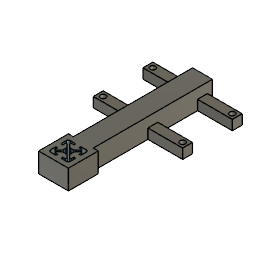
Spiegel Houder (Autodesk Fusion 360 design; units mm, degrees)
part number: 2026-06-02-17-48-06-429
Autodesk Fusion 360 part; units mm, degrees
note: some values were not read from the file. Set by a fixed rule: which sketch regions a step uses.
sketch "Item profile" plane through (0, 0, 0) normal (0, 0, 1) x (1, 0, 0)
  line L0 (2.5199, -9.1957) -> (2.5199, -8.4981)
  spline S0 degree 3 poles (2.5199, -8.4981) (2.5279, -8.3313) (2.6117, -8.22) (2.8181, -8.1997) knots 0 0 0 0 1 1 1 1
  line L1 (2.8181, -8.1997) -> (4.9343, -8.1997)
  spline S1 degree 3 poles (4.9343, -8.1997) (5.7717, -8.1578) (5.9819, -7.2415) (5.5227, -6.7803) knots 0 0 0 0 1 1 1 1
  line L2 (5.5227, -6.7803) -> (3.2736, -4.5302)
  spline S2 degree 3 poles (3.2736, -4.5302) (2.3958, -3.7139) (1.5457, -3.6474) (1.1575, -3.6552) knots 0 0 0 0 1 1 1 1
  line L3 (1.1575, -3.6552) -> (-1.1199, -3.6552)
  spline S3 degree 3 poles (-1.1199, -3.6552) (-1.5201, -3.6474) (-2.3702, -3.7139) (-3.2481, -4.5302) knots 0 0 0 0 1 1 1 1
  line L4 (-3.2481, -4.5302) -> (-5.4972, -6.7803)
  spline S4 degree 3 poles (-5.4972, -6.7803) (-5.9564, -7.2415) (-5.7462, -8.1578) (-4.9087, -8.1997) knots 0 0 0 0 1 1 1 1
  line L5 (-4.9087, -8.1997) -> (-2.7926, -8.1997)
  spline S5 degree 3 poles (-2.7926, -8.1997) (-2.5862, -8.22) (-2.5027, -8.3313) (-2.4943, -8.4981) knots 0 0 0 0 1 1 1 1
  line L6 (-2.4943, -8.4981) -> (-2.4943, -9.1957)
  spline S6 degree 3 poles (-2.4943, -9.1957) (-2.5003, -9.6292) (-2.8228, -9.9778) (-3.2985, -9.9941) knots 0 0 0 0 1 1 1 1
  line L7 (-3.2985, -9.9941) -> (-7.9963, -9.9941)
  spline S7 degree 3 poles (-7.9963, -9.9941) (-9.0202, -10.009) (-10.0068, -9.1289) (-9.9915, -7.994) knots 0 0 0 0 1 1 1 1
  line L8 (-9.9915, -7.994) -> (-9.9915, -3.3004)
  spline S8 degree 3 poles (-9.9915, -3.3004) (-9.9752, -2.8306) (-9.6268, -2.5081) (-9.1934, -2.502) knots 0 0 0 0 1 1 1 1
  line L9 (-9.1934, -2.502) -> (-8.4961, -2.502)
  spline S9 degree 3 poles (-8.4961, -2.502) (-8.3294, -2.5103) (-8.2182, -2.5938) (-8.1978, -2.8003) knots 0 0 0 0 1 1 1 1
  line L10 (-8.1978, -2.8003) -> (-8.1978, -4.9173)
  spline S10 degree 3 poles (-8.1978, -4.9173) (-8.1559, -5.7552) (-7.24, -5.9654) (-6.779, -5.5061) knots 0 0 0 0 1 1 1 1
  line L11 (-6.779, -5.5061) -> (-4.5299, -3.256)
  spline S11 degree 3 poles (-4.5299, -3.256) (-3.7139, -2.3778) (-3.6474, -1.5274) (-3.6552, -1.139) knots 0 0 0 0 1 1 1 1
  line L12 (-3.6552, -1.139) -> (-3.6552, 1.1393)
  spline S12 degree 3 poles (-3.6552, 1.1393) (-3.6472, 1.5397) (-3.7138, 2.3901) (-4.5299, 3.2683) knots 0 0 0 0 1 1 1 1
  line L13 (-4.5299, 3.2683) -> (-6.779, 5.5184)
  spline S13 degree 3 poles (-6.779, 5.5184) (-7.24, 5.9777) (-8.1559, 5.7675) (-8.1978, 4.9297) knots 0 0 0 0 1 1 1 1
  line L14 (-8.1978, 4.9297) -> (-8.1978, 2.8127)
  spline S14 degree 3 poles (-8.1978, 2.8127) (-8.2181, 2.6062) (-8.3294, 2.5226) (-8.4961, 2.5143) knots 0 0 0 0 1 1 1 1
  line L15 (-8.4961, 2.5143) -> (-9.1934, 2.5143)
  spline S15 degree 3 poles (-9.1934, 2.5143) (-9.6267, 2.5204) (-9.9752, 2.8429) (-9.9915, 3.3085) knots 0 0 0 0 1 1 1 1
  line L16 (-9.9915, 3.3085) -> (-9.9915, 7.9981)
  spline S16 degree 3 poles (-9.9915, 7.9981) (-10.0064, 9.0224) (-9.1267, 10.0093) (-7.9922, 9.9941) knots 0 0 0 0 1 1 1 1
  line L17 (-7.9922, 9.9941) -> (-3.3005, 9.9941)
  spline S17 degree 3 poles (-3.3005, 9.9941) (-2.8309, 9.9778) (-2.5086, 9.6292) (-2.5024, 9.1957) knots 0 0 0 0 1 1 1 1
  line L18 (-2.5024, 9.1957) -> (-2.5024, 8.4981)
  spline S18 degree 3 poles (-2.5024, 8.4981) (-2.5104, 8.3313) (-2.5943, 8.22) (-2.8007, 8.1997) knots 0 0 0 0 1 1 1 1
  line L19 (-2.8007, 8.1997) -> (-4.9168, 8.1997)
  spline S19 degree 3 poles (-4.9168, 8.1997) (-5.7543, 8.1578) (-5.9645, 7.2415) (-5.5053, 6.7803) knots 0 0 0 0 1 1 1 1
  line L20 (-5.5053, 6.7803) -> (-3.2562, 4.5302)
  spline S20 degree 3 poles (-3.2562, 4.5302) (-2.3783, 3.7139) (-1.5283, 3.6474) (-1.14, 3.6552) knots 0 0 0 0 1 1 1 1
  line L21 (-1.14, 3.6552) -> (1.1373, 3.6552)
  spline S21 degree 3 poles (1.1373, 3.6552) (1.5376, 3.6474) (2.3877, 3.7139) (3.2655, 4.5302) knots 0 0 0 0 1 1 1 1
  line L22 (3.2655, 4.5302) -> (5.5147, 6.7803)
  spline S22 degree 3 poles (5.5147, 6.7803) (5.9738, 7.2414) (5.7636, 8.1577) (4.9262, 8.1996) knots 0 0 0 0 1 1 1 1
  line L23 (4.9262, 8.1996) -> (2.81, 8.1996)
  spline S23 degree 3 poles (2.81, 8.1996) (2.6036, 8.22) (2.5201, 8.3312) (2.5118, 8.498) knots 0 0 0 0 1 1 1 1
  line L24 (2.5118, 8.498) -> (2.5118, 9.1956)
  spline S24 degree 3 poles (2.5118, 9.1956) (2.5178, 9.6292) (2.8403, 9.9778) (3.3159, 9.994) knots 0 0 0 0 1 1 1 1
  line L25 (3.3159, 9.994) -> (8.0137, 9.9941)
  spline S25 degree 3 poles (8.0137, 9.9941) (9.0376, 10.009) (10.0242, 9.1289) (10.0089, 7.994) knots 0 0 0 0 1 1 1 1
  line L26 (10.0089, 7.994) -> (10.0089, 3.3004)
  spline S26 degree 3 poles (10.0089, 3.3004) (9.9927, 2.8306) (9.6442, 2.5081) (9.2109, 2.502) knots 0 0 0 0 1 1 1 1
  line L27 (9.2109, 2.502) -> (8.5136, 2.502)
  spline S27 degree 3 poles (8.5136, 2.502) (8.3468, 2.5103) (8.2356, 2.5938) (8.2153, 2.8003) knots 0 0 0 0 1 1 1 1
  line L28 (8.2153, 2.8003) -> (8.2153, 4.9173)
  spline S28 degree 3 poles (8.2153, 4.9173) (8.1734, 5.7551) (7.2575, 5.9654) (6.7965, 5.5061) knots 0 0 0 0 1 1 1 1
  line L29 (6.7965, 5.5061) -> (4.5473, 3.256)
  spline S29 degree 3 poles (4.5473, 3.256) (3.7313, 2.3778) (3.6649, 1.5274) (3.6727, 1.139) knots 0 0 0 0 1 1 1 1
  line L30 (3.6727, 1.139) -> (3.6727, -1.1392)
  spline S30 degree 3 poles (3.6727, -1.1392) (3.6646, -1.5397) (3.7312, -2.3901) (4.5473, -3.2683) knots 0 0 0 0 1 1 1 1
  line L31 (4.5473, -3.2683) -> (6.7964, -5.5184)
  spline S31 degree 3 poles (6.7964, -5.5184) (7.2574, -5.9777) (8.1734, -5.7675) (8.2153, -4.9296) knots 0 0 0 0 1 1 1 1
  line L32 (8.2153, -4.9296) -> (8.2153, -2.8126)
  spline S32 degree 3 poles (8.2153, -2.8126) (8.2356, -2.6061) (8.3468, -2.5226) (8.5135, -2.5143) knots 0 0 0 0 1 1 1 1
  line L33 (8.5135, -2.5143) -> (9.2108, -2.5143)
  spline S33 degree 3 poles (9.2108, -2.5143) (9.6442, -2.5204) (9.9927, -2.8429) (10.0089, -3.3127) knots 0 0 0 0 1 1 1 1
  line L34 (10.0089, -3.3127) -> (10.0089, -8.0063)
  spline S34 degree 3 poles (10.0089, -8.0063) (10.0242, -9.1412) (9.0376, -10.0213) (8.0137, -10.0064) knots 0 0 0 0 1 1 1 1
  line L35 (8.0137, -10.0064) -> (3.32, -10.0002)
  spline S35 degree 3 poles (3.32, -10.0002) (2.8483, -9.9778) (2.526, -9.6292) (2.5199, -9.1957) knots 0 0 0 0 1 1 1 1
  circle A0 centre (0, 0) radius 3.6552 construction
  constraint tangent L3 A0
  constraint tangent L12 A0
  constraint tangent L21 A0
  constraint coincident A0.centre origin
sketch "Body profile" plane through (0, 0, 0) normal (0, 0, 1) x (1, 0, 0)
  line L0 (15, 15) -> (-15, 15)
  line L1 (-15, 15) -> (-15, -15)
  line L2 (-15, -15) -> (15, -15)
  line L3 (15, -15) -> (15, 15)
  line L4 (15, 15) -> (-15, -15) construction
  line L5 (-15, 15) -> (15, -15) construction
  dimension "d1" = 30
  dimension "d2" = 30
  constraint horizontal L0
  constraint perpendicular L0 L1
  constraint parallel L0 L2
  constraint parallel L1 L3
  constraint coincident L4 origin
  constraint coincident L5 origin
  measures "d1" distance of L1.end L2.end
  measures "d2" distance of L0.end L1.end
extrude "Extrude1" add sketch "Body profile" along normal blind 20
extrude "Extrude13" cut sketch "Item profile" along normal blind 20
sketch "Sketch11" plane through (0, 15, 0) normal (0, 1, 0) x (1, 0, 0)
  line L0 (10, 0) -> (-10, 0) construction
  line L1 (10, 0) -> (-10, 0)
  line L2 (-10, 0) -> (-10, -20)
  line L3 (-10, -20) -> (10, -20)
  line L4 (10, -20) -> (10, 0)
  line L5 (15, 0) -> (-15, 0)
  line L6 (-15, 0) -> (-15, -20)
  line L7 (-15, -20) -> (15, -20)
  line L8 (15, -20) -> (15, 0)
  dimension "d60" = 20
  dimension "d61" = 20
  constraint horizontal L1
  constraint vertical L2
  constraint horizontal L3
  constraint vertical L4
  constraint coincident L0.start L1.start
  measures "d60" distance of L0.start L0.end
  measures "d61" distance of L0.start L3.end
extrude "Extrude9" add sketch "Sketch11" along normal blind 120 contours L1 L2 L3 L4 L5 L7
sketch "Sketch12" plane through (-10, 0, 0) normal (-1, 0, 0) x (0, -1, 0)
  line L0 (-15, 0) -> (-15, 20)
  line L1 (-130, 0) -> (-120, 0)
  line L2 (-120, 0) -> (-120, 10)
  line L3 (-120, 10) -> (-130, 10)
  line L4 (-130, 10) -> (-130, 0)
  line L5 (-80, 0) -> (-70, 0)
  line L6 (-70, 0) -> (-70, 10)
  line L7 (-70, 10) -> (-80, 10)
  line L8 (-80, 10) -> (-80, 0)
  line L9 (-15, 0) -> (-15, 20)
  line L10 (-15, 20) -> (-135, 20)
  line L11 (-135, 20) -> (-135, 0)
  line L12 (-135, 0) -> (-15, 0)
  dimension "d65" = 10
  dimension "d66" = 10
  dimension "d67" = 10
  dimension "d68" = 10
  dimension "d69" = 60
  dimension "d104" = 5
  constraint horizontal L1
  constraint vertical L2
  constraint horizontal L3
  constraint vertical L4
  constraint horizontal L5
  constraint vertical L6
  constraint horizontal L7
  constraint vertical L8
  constraint collinear L1 L12
  constraint collinear L5 L12
  measures "d65" distance of L1.start L1.end
  measures "d66" distance of L1.start L3.end
  measures "d67" distance of L5.start L5.end
  measures "d68" distance of L5.start L7.end
  measures "d69" distance of L4 L6
  measures "d104" distance of L4 L11
extrude "Extrude10" add sketch "Sketch12" along normal blind 35 contours L5 L6 L7 L8 L12 | L1 L2 L3 L4 L12
sketch "Sketch14" plane through (0, 0, 10) normal (0, 0, 1) x (-1, 0, 0)
  line L0 (10, -80) -> (45, -80)
  line L1 (45, -80) -> (45, -70)
  line L2 (45, -70) -> (10, -70)
  line L3 (45, -75) -> (35, -75) construction
  circle A0 centre (40, -75) radius 2.75
  circle A1 centre (40, -75) radius 1.5
  line L4 (10, -70) -> (10, -80)
  dimension "d78" = 10
  dimension "d79" = 5.5
  dimension "d80" = 3
  constraint midpoint L1 L3.start
  constraint perpendicular L1 L3
  constraint midpoint L3 A0.centre
  constraint concentric A0 A1
  measures "d78" distance of L3.start L3.end
  measures "d79" diameter of A0
  measures "d80" diameter of A1
extrude "Extrude11" cut sketch "Sketch14" against normal blind 10 contours A1
extrude "Extrude12" cut sketch "Sketch14" against normal blind 8 contours A0
pattern_linear "R-Pattern1" count 2 spacing 50 along (0, 1, 0) of "Extrude11", "Extrude12"
mirror "Mirror3" about plane through (0, 0, 0) normal (1, 0, 0) of "Extrude10", "Extrude11", "Extrude12", "R-Pattern1"
sketch "Sketch13" plane through (0, 0, 0) normal (0, 0, -1) x (1, 0, 0)
  line L0 (-10, -70) -> (-45, -70)
  line L1 (-45, -70) -> (-45, -80)
  line L2 (-45, -80) -> (-10, -80)
  line L3 (-10, -120) -> (-45, -120)
  line L4 (-45, -120) -> (-45, -130)
  line L5 (-45, -130) -> (-10, -130)
  line L6 (-10, -135) -> (10, -135)
  line L7 (10, -130) -> (45, -130)
  line L8 (45, -130) -> (45, -120)
  line L9 (45, -120) -> (10, -120)
  line L10 (10, -80) -> (45, -80)
  line L11 (45, -80) -> (45, -70)
  line L12 (45, -70) -> (10, -70)
  line L13 (-10, -125.1421) -> (10, -125.1421) construction
  line L14 (-35, -160.1421) -> (35, -160.1421) construction
  line L15 (35, -160.1421) -> (35, -90.1421) construction
  line L16 (35, -90.1421) -> (-35, -90.1421) construction
  line L17 (-35, -90.1421) -> (-35, -160.1421) construction
  line L18 (-35, -160.1421) -> (35, -90.1421) construction
  line L19 (35, -160.1421) -> (-35, -90.1421) construction
  circle A0 centre (-40, -125) radius 1.5
  circle A1 centre (-40, -75) radius 1.5
  circle A2 centre (40, -125) radius 1.5
  circle A3 centre (40, -75) radius 1.5
  spline S0 degree 3 poles (2.5199, 9.1957) (2.526, 9.6292) (2.8483, 9.9778) (3.32, 10.0002) knots -1 -1 -1 -1 0 0 0 0
  line L20 (3.32, 10.0002) -> (8.0137, 10.0064)
  spline S1 degree 3 poles (8.0137, 10.0064) (9.0376, 10.0213) (10.0242, 9.1412) (10.0089, 8.0063) knots -1 -1 -1 -1 0 0 0 0
  line L21 (10.0089, 8.0063) -> (10.0089, 3.3127)
  spline S2 degree 3 poles (10.0089, 3.3127) (9.9927, 2.8429) (9.6442, 2.5204) (9.2108, 2.5143) knots -1 -1 -1 -1 0 0 0 0
  line L22 (9.2108, 2.5143) -> (8.5135, 2.5143)
  spline S3 degree 3 poles (8.5135, 2.5143) (8.3468, 2.5226) (8.2356, 2.6061) (8.2153, 2.8126) knots -1 -1 -1 -1 0 0 0 0
  line L23 (8.2153, 2.8126) -> (8.2153, 4.9296)
  spline S4 degree 3 poles (8.2153, 4.9296) (8.1734, 5.7675) (7.2574, 5.9777) (6.7964, 5.5184) knots -1 -1 -1 -1 0 0 0 0
  line L24 (6.7964, 5.5184) -> (4.5473, 3.2683)
  spline S5 degree 3 poles (4.5473, 3.2683) (3.7312, 2.3901) (3.6646, 1.5397) (3.6727, 1.1392) knots -1 -1 -1 -1 0 0 0 0
  line L25 (3.6727, 1.1392) -> (3.6727, -1.139)
  spline S6 degree 3 poles (3.6727, -1.139) (3.6649, -1.5274) (3.7313, -2.3778) (4.5473, -3.256) knots -1 -1 -1 -1 0 0 0 0
  line L26 (4.5473, -3.256) -> (6.7965, -5.5061)
  spline S7 degree 3 poles (6.7965, -5.5061) (7.2575, -5.9654) (8.1734, -5.7551) (8.2153, -4.9173) knots -1 -1 -1 -1 0 0 0 0
  line L27 (8.2153, -4.9173) -> (8.2153, -2.8003)
  spline S8 degree 3 poles (8.2153, -2.8003) (8.2356, -2.5938) (8.3468, -2.5103) (8.5136, -2.502) knots -1 -1 -1 -1 0 0 0 0
  line L28 (8.5136, -2.502) -> (9.2109, -2.502)
  spline S9 degree 3 poles (9.2109, -2.502) (9.6442, -2.5081) (9.9927, -2.8306) (10.0089, -3.3004) knots -1 -1 -1 -1 0 0 0 0
  line L29 (10.0089, -3.3004) -> (10.0089, -7.994)
  spline S10 degree 3 poles (10.0089, -7.994) (10.0242, -9.1289) (9.0376, -10.009) (8.0137, -9.9941) knots -1 -1 -1 -1 0 0 0 0
  line L30 (8.0137, -9.9941) -> (3.3159, -9.994)
  spline S11 degree 3 poles (3.3159, -9.994) (2.8403, -9.9778) (2.5178, -9.6292) (2.5118, -9.1956) knots -1 -1 -1 -1 0 0 0 0
  line L31 (2.5118, -9.1956) -> (2.5118, -8.498)
  spline S12 degree 3 poles (2.5118, -8.498) (2.5201, -8.3312) (2.6036, -8.22) (2.81, -8.1996) knots -1 -1 -1 -1 0 0 0 0
  line L32 (2.81, -8.1996) -> (4.9262, -8.1996)
  spline S13 degree 3 poles (4.9262, -8.1996) (5.7636, -8.1577) (5.9738, -7.2414) (5.5147, -6.7803) knots -1 -1 -1 -1 0 0 0 0
  line L33 (5.5147, -6.7803) -> (3.2655, -4.5302)
  spline S14 degree 3 poles (3.2655, -4.5302) (2.3877, -3.7139) (1.5376, -3.6474) (1.1373, -3.6552) knots -1 -1 -1 -1 0 0 0 0
  line L34 (1.1373, -3.6552) -> (-1.14, -3.6552)
  spline S15 degree 3 poles (-1.14, -3.6552) (-1.5283, -3.6474) (-2.3783, -3.7139) (-3.2562, -4.5302) knots -1 -1 -1 -1 0 0 0 0
  line L35 (-3.2562, -4.5302) -> (-5.5053, -6.7803)
  spline S16 degree 3 poles (-5.5053, -6.7803) (-5.9645, -7.2415) (-5.7543, -8.1578) (-4.9168, -8.1997) knots -1 -1 -1 -1 0 0 0 0
  line L36 (-4.9168, -8.1997) -> (-2.8007, -8.1997)
  spline S17 degree 3 poles (-2.8007, -8.1997) (-2.5943, -8.22) (-2.5104, -8.3313) (-2.5024, -8.4981) knots -1 -1 -1 -1 0 0 0 0
  line L37 (-2.5024, -8.4981) -> (-2.5024, -9.1957)
  spline S18 degree 3 poles (-2.5024, -9.1957) (-2.5086, -9.6292) (-2.8309, -9.9778) (-3.3005, -9.9941) knots -1 -1 -1 -1 0 0 0 0
  line L38 (-3.3005, -9.9941) -> (-7.9922, -9.9941)
  spline S19 degree 3 poles (-7.9922, -9.9941) (-9.1267, -10.0093) (-10.0064, -9.0224) (-9.9915, -7.9981) knots -1 -1 -1 -1 0 0 0 0
  line L39 (-9.9915, -7.9981) -> (-9.9915, -3.3085)
  spline S20 degree 3 poles (-9.9915, -3.3085) (-9.9752, -2.8429) (-9.6267, -2.5204) (-9.1934, -2.5143) knots -1 -1 -1 -1 0 0 0 0
  line L40 (-9.1934, -2.5143) -> (-8.4961, -2.5143)
  spline S21 degree 3 poles (-8.4961, -2.5143) (-8.3294, -2.5226) (-8.2181, -2.6062) (-8.1978, -2.8127) knots -1 -1 -1 -1 0 0 0 0
  line L41 (-8.1978, -2.8127) -> (-8.1978, -4.9297)
  spline S22 degree 3 poles (-8.1978, -4.9297) (-8.1559, -5.7675) (-7.24, -5.9777) (-6.779, -5.5184) knots -1 -1 -1 -1 0 0 0 0
  line L42 (-6.779, -5.5184) -> (-4.5299, -3.2683)
  spline S23 degree 3 poles (-4.5299, -3.2683) (-3.7138, -2.3901) (-3.6472, -1.5397) (-3.6552, -1.1393) knots -1 -1 -1 -1 0 0 0 0
  line L43 (-3.6552, -1.1393) -> (-3.6552, 1.139)
  spline S24 degree 3 poles (-3.6552, 1.139) (-3.6474, 1.5274) (-3.7139, 2.3778) (-4.5299, 3.256) knots -1 -1 -1 -1 0 0 0 0
  line L44 (-4.5299, 3.256) -> (-6.779, 5.5061)
  spline S25 degree 3 poles (-6.779, 5.5061) (-7.24, 5.9654) (-8.1559, 5.7552) (-8.1978, 4.9173) knots -1 -1 -1 -1 0 0 0 0
  line L45 (-8.1978, 4.9173) -> (-8.1978, 2.8003)
  spline S26 degree 3 poles (-8.1978, 2.8003) (-8.2182, 2.5938) (-8.3294, 2.5103) (-8.4961, 2.502) knots -1 -1 -1 -1 0 0 0 0
  line L46 (-8.4961, 2.502) -> (-9.1934, 2.502)
  spline S27 degree 3 poles (-9.1934, 2.502) (-9.6268, 2.5081) (-9.9752, 2.8306) (-9.9915, 3.3004) knots -1 -1 -1 -1 0 0 0 0
  line L47 (-9.9915, 3.3004) -> (-9.9915, 7.994)
  spline S28 degree 3 poles (-9.9915, 7.994) (-10.0068, 9.1289) (-9.0202, 10.009) (-7.9963, 9.9941) knots -1 -1 -1 -1 0 0 0 0
  line L48 (-7.9963, 9.9941) -> (-3.2985, 9.9941)
  spline S29 degree 3 poles (-3.2985, 9.9941) (-2.8228, 9.9778) (-2.5003, 9.6292) (-2.4943, 9.1957) knots -1 -1 -1 -1 0 0 0 0
  line L49 (-2.4943, 9.1957) -> (-2.4943, 8.4981)
  spline S30 degree 3 poles (-2.4943, 8.4981) (-2.5027, 8.3313) (-2.5862, 8.22) (-2.7926, 8.1997) knots -1 -1 -1 -1 0 0 0 0
  line L50 (-2.7926, 8.1997) -> (-4.9087, 8.1997)
  spline S31 degree 3 poles (-4.9087, 8.1997) (-5.7462, 8.1578) (-5.9564, 7.2415) (-5.4972, 6.7803) knots -1 -1 -1 -1 0 0 0 0
  line L51 (-5.4972, 6.7803) -> (-3.2481, 4.5302)
  spline S32 degree 3 poles (-3.2481, 4.5302) (-2.3702, 3.7139) (-1.5201, 3.6474) (-1.1199, 3.6552) knots -1 -1 -1 -1 0 0 0 0
  line L52 (-1.1199, 3.6552) -> (1.1575, 3.6552)
  spline S33 degree 3 poles (1.1575, 3.6552) (1.5457, 3.6474) (2.3958, 3.7139) (3.2736, 4.5302) knots -1 -1 -1 -1 0 0 0 0
  line L53 (3.2736, 4.5302) -> (5.5227, 6.7803)
  spline S34 degree 3 poles (5.5227, 6.7803) (5.9819, 7.2415) (5.7717, 8.1578) (4.9343, 8.1997) knots -1 -1 -1 -1 0 0 0 0
  line L54 (4.9343, 8.1997) -> (2.8181, 8.1997)
  spline S35 degree 3 poles (2.8181, 8.1997) (2.6117, 8.22) (2.5279, 8.3313) (2.5199, 8.4981) knots -1 -1 -1 -1 0 0 0 0
  line L55 (2.5199, 8.4981) -> (2.5199, 9.1957)
  line L56 (15, -15) -> (15, 15)
  line L57 (15, 15) -> (-15, 15)
  line L58 (-15, 15) -> (-15, -15)
  line L59 (-15, -15) -> (-10, -15)
  line L60 (-10, -15) -> (-10, -70)
  line L61 (-10, -80) -> (-10, -120)
  line L62 (-10, -130) -> (-10, -135)
  line L63 (10, -135) -> (10, -130)
  line L64 (10, -120) -> (10, -80)
  line L65 (10, -70) -> (10, -15)
  line L66 (10, -15) -> (15, -15)
  point P0 (0, -125.1421)
  dimension "d76" = 70
  dimension "d77" = 70
  constraint horizontal L14
  constraint perpendicular L14 L15
  constraint parallel L14 L16
  constraint parallel L15 L17
  constraint coincident L18 P0
  constraint coincident L19 P0
  constraint midpoint L13 P0
  measures "d76" distance of L15.end L16.end
  measures "d77" distance of L14.end L15.end
sketch "Sketch15" plane through (0, 0, 20) normal (0, 0, 1) x (-1, 0, 0)
  spline S0 degree 3 poles (-3.32, 10.0002) (-2.8483, 9.9778) (-2.526, 9.6292) (-2.5199, 9.1957) knots 0 0 0 0 1 1 1 1
  line L0 (-2.5199, 9.1957) -> (-2.5199, 8.4981)
  spline S1 degree 3 poles (-2.5199, 8.4981) (-2.5279, 8.3313) (-2.6117, 8.22) (-2.8181, 8.1997) knots 0 0 0 0 1 1 1 1
  line L1 (-2.8181, 8.1997) -> (-4.9343, 8.1997)
  spline S2 degree 3 poles (-4.9343, 8.1997) (-5.7717, 8.1578) (-5.9819, 7.2415) (-5.5227, 6.7803) knots 0 0 0 0 1 1 1 1
  line L2 (-5.5227, 6.7803) -> (-3.2736, 4.5302)
  spline S3 degree 3 poles (-3.2736, 4.5302) (-2.3958, 3.7139) (-1.5457, 3.6474) (-1.1575, 3.6552) knots 0 0 0 0 1 1 1 1
  line L3 (-1.1575, 3.6552) -> (1.1199, 3.6552)
  spline S4 degree 3 poles (1.1199, 3.6552) (1.5201, 3.6474) (2.3702, 3.7139) (3.2481, 4.5302) knots 0 0 0 0 1 1 1 1
  line L4 (3.2481, 4.5302) -> (5.4972, 6.7803)
  spline S5 degree 3 poles (5.4972, 6.7803) (5.9564, 7.2415) (5.7462, 8.1578) (4.9087, 8.1997) knots 0 0 0 0 1 1 1 1
  line L5 (4.9087, 8.1997) -> (2.7926, 8.1997)
  spline S6 degree 3 poles (2.7926, 8.1997) (2.5862, 8.22) (2.5027, 8.3313) (2.4943, 8.4981) knots 0 0 0 0 1 1 1 1
  line L6 (2.4943, 8.4981) -> (2.4943, 9.1957)
  spline S7 degree 3 poles (2.4943, 9.1957) (2.5003, 9.6292) (2.8228, 9.9778) (3.2985, 9.9941) knots 0 0 0 0 1 1 1 1
  line L7 (3.2985, 9.9941) -> (7.9963, 9.9941)
  spline S8 degree 3 poles (7.9963, 9.9941) (9.0202, 10.009) (10.0068, 9.1289) (9.9915, 7.994) knots 0 0 0 0 1 1 1 1
  line L8 (9.9915, 7.994) -> (9.9915, 3.3004)
  spline S9 degree 3 poles (9.9915, 3.3004) (9.9752, 2.8306) (9.6268, 2.5081) (9.1934, 2.502) knots 0 0 0 0 1 1 1 1
  line L9 (9.1934, 2.502) -> (8.4961, 2.502)
  spline S10 degree 3 poles (8.4961, 2.502) (8.3294, 2.5103) (8.2182, 2.5938) (8.1978, 2.8003) knots 0 0 0 0 1 1 1 1
  line L10 (8.1978, 2.8003) -> (8.1978, 4.9173)
  spline S11 degree 3 poles (8.1978, 4.9173) (8.1559, 5.7552) (7.24, 5.9654) (6.779, 5.5061) knots 0 0 0 0 1 1 1 1
  line L11 (6.779, 5.5061) -> (4.5299, 3.256)
  spline S12 degree 3 poles (4.5299, 3.256) (3.7139, 2.3778) (3.6474, 1.5274) (3.6552, 1.139) knots 0 0 0 0 1 1 1 1
  line L12 (3.6552, 1.139) -> (3.6552, -1.1393)
  spline S13 degree 3 poles (3.6552, -1.1393) (3.6472, -1.5397) (3.7138, -2.3901) (4.5299, -3.2683) knots 0 0 0 0 1 1 1 1
  line L13 (4.5299, -3.2683) -> (6.779, -5.5184)
  spline S14 degree 3 poles (6.779, -5.5184) (7.24, -5.9777) (8.1559, -5.7675) (8.1978, -4.9297) knots 0 0 0 0 1 1 1 1
  line L14 (8.1978, -4.9297) -> (8.1978, -2.8127)
  spline S15 degree 3 poles (8.1978, -2.8127) (8.2181, -2.6062) (8.3294, -2.5226) (8.4961, -2.5143) knots 0 0 0 0 1 1 1 1
  line L15 (8.4961, -2.5143) -> (9.1934, -2.5143)
  spline S16 degree 3 poles (9.1934, -2.5143) (9.6267, -2.5204) (9.9752, -2.8429) (9.9915, -3.3085) knots 0 0 0 0 1 1 1 1
  line L16 (9.9915, -3.3085) -> (9.9915, -7.9981)
  spline S17 degree 3 poles (9.9915, -7.9981) (10.0064, -9.0224) (9.1267, -10.0093) (7.9922, -9.9941) knots 0 0 0 0 1 1 1 1
  line L17 (7.9922, -9.9941) -> (3.3005, -9.9941)
  spline S18 degree 3 poles (3.3005, -9.9941) (2.8309, -9.9778) (2.5086, -9.6292) (2.5024, -9.1957) knots 0 0 0 0 1 1 1 1
  line L18 (2.5024, -9.1957) -> (2.5024, -8.4981)
  spline S19 degree 3 poles (2.5024, -8.4981) (2.5104, -8.3313) (2.5943, -8.22) (2.8007, -8.1997) knots 0 0 0 0 1 1 1 1
  line L19 (2.8007, -8.1997) -> (4.9168, -8.1997)
  spline S20 degree 3 poles (4.9168, -8.1997) (5.7543, -8.1578) (5.9645, -7.2415) (5.5053, -6.7803) knots 0 0 0 0 1 1 1 1
  line L20 (5.5053, -6.7803) -> (3.2562, -4.5302)
  spline S21 degree 3 poles (3.2562, -4.5302) (2.3783, -3.7139) (1.5283, -3.6474) (1.14, -3.6552) knots 0 0 0 0 1 1 1 1
  line L21 (1.14, -3.6552) -> (-1.1373, -3.6552)
  spline S22 degree 3 poles (-1.1373, -3.6552) (-1.5376, -3.6474) (-2.3877, -3.7139) (-3.2655, -4.5302) knots 0 0 0 0 1 1 1 1
  line L22 (-3.2655, -4.5302) -> (-5.5147, -6.7803)
  spline S23 degree 3 poles (-5.5147, -6.7803) (-5.9738, -7.2414) (-5.7636, -8.1577) (-4.9262, -8.1996) knots 0 0 0 0 1 1 1 1
  line L23 (-4.9262, -8.1996) -> (-2.81, -8.1996)
  spline S24 degree 3 poles (-2.81, -8.1996) (-2.6036, -8.22) (-2.5201, -8.3312) (-2.5118, -8.498) knots 0 0 0 0 1 1 1 1
  line L24 (-2.5118, -8.498) -> (-2.5118, -9.1956)
  spline S25 degree 3 poles (-2.5118, -9.1956) (-2.5178, -9.6292) (-2.8403, -9.9778) (-3.3159, -9.994) knots 0 0 0 0 1 1 1 1
  line L25 (-3.3159, -9.994) -> (-8.0137, -9.9941)
  spline S26 degree 3 poles (-8.0137, -9.9941) (-9.0376, -10.009) (-10.0242, -9.1289) (-10.0089, -7.994) knots 0 0 0 0 1 1 1 1
  line L26 (-10.0089, -7.994) -> (-10.0089, -3.3004)
  spline S27 degree 3 poles (-10.0089, -3.3004) (-9.9927, -2.8306) (-9.6442, -2.5081) (-9.2109, -2.502) knots 0 0 0 0 1 1 1 1
  line L27 (-9.2109, -2.502) -> (-8.5136, -2.502)
  spline S28 degree 3 poles (-8.5136, -2.502) (-8.3468, -2.5103) (-8.2356, -2.5938) (-8.2153, -2.8003) knots 0 0 0 0 1 1 1 1
  line L28 (-8.2153, -2.8003) -> (-8.2153, -4.9173)
  spline S29 degree 3 poles (-8.2153, -4.9173) (-8.1734, -5.7551) (-7.2575, -5.9654) (-6.7965, -5.5061) knots 0 0 0 0 1 1 1 1
  line L29 (-6.7965, -5.5061) -> (-4.5473, -3.256)
  spline S30 degree 3 poles (-4.5473, -3.256) (-3.7313, -2.3778) (-3.6649, -1.5274) (-3.6727, -1.139) knots 0 0 0 0 1 1 1 1
  line L30 (-3.6727, -1.139) -> (-3.6727, 1.1392)
  spline S31 degree 3 poles (-3.6727, 1.1392) (-3.6646, 1.5397) (-3.7312, 2.3901) (-4.5473, 3.2683) knots 0 0 0 0 1 1 1 1
  line L31 (-4.5473, 3.2683) -> (-6.7964, 5.5184)
  spline S32 degree 3 poles (-6.7964, 5.5184) (-7.2574, 5.9777) (-8.1734, 5.7675) (-8.2153, 4.9296) knots 0 0 0 0 1 1 1 1
  line L32 (-8.2153, 4.9296) -> (-8.2153, 2.8126)
  spline S33 degree 3 poles (-8.2153, 2.8126) (-8.2356, 2.6061) (-8.3468, 2.5226) (-8.5135, 2.5143) knots 0 0 0 0 1 1 1 1
  line L33 (-8.5135, 2.5143) -> (-9.2108, 2.5143)
  spline S34 degree 3 poles (-9.2108, 2.5143) (-9.6442, 2.5204) (-9.9927, 2.8429) (-10.0089, 3.3127) knots 0 0 0 0 1 1 1 1
  line L34 (-10.0089, 3.3127) -> (-10.0089, 8.0063)
  spline S35 degree 3 poles (-10.0089, 8.0063) (-10.0242, 9.1412) (-9.0376, 10.0213) (-8.0137, 10.0064) knots 0 0 0 0 1 1 1 1
  line L35 (-8.0137, 10.0064) -> (-3.32, 10.0002)
  line L36 (-15, 15) -> (-15, -15)
  line L37 (-15, -15) -> (-10, -15)
  line L38 (-10, -15) -> (-10, -135)
  line L39 (-10, -135) -> (10, -135)
  line L40 (10, -135) -> (10, -15)
  line L41 (10, -15) -> (15, -15)
  line L42 (15, -15) -> (15, 15)
  line L43 (15, 15) -> (-15, 15)
scale "Scale2" factor 1.008 about (-10, 70, 0) bodies 1
